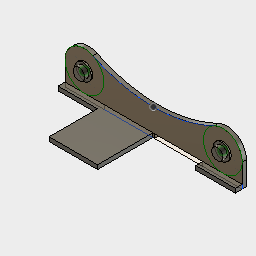
spoolholder (Autodesk Fusion 360 design; units mm, degrees)
Autodesk Fusion 360 part; units mm, degrees
sketch "Sketch1" plane through (0, 0, 0) normal (0, 0, 1) x (1, 0, 0)
  circle A0 centre (-50, 0) radius 4.1
  circle A1 centre (50, 0) radius 4.1
  circle A2 centre (50, 0) radius 14
  circle A3 centre (50, 0) radius 6
  circle A4 centre (-50, 0) radius 14
  circle A5 centre (-50, 0) radius 6
  line L0 (-64, -14) -> (64, -14)
  line L1 (-64, 0) -> (-64, -14)
  line L2 (64, 0) -> (64, -14)
  arc A6 (-43.8635, 12.5835) -> (43.8635, 12.5835) centre (0, 102.5297) ccw
  line L3 (-64, -14) -> (64, -14)
  line L4 (64, -14) -> (64, -17)
  line L5 (64, -17) -> (-64, -17)
  line L6 (-64, -17) -> (-64, -14)
  line L7 (0.5, -14) -> (35.5, -14)
  line L8 (35.5, -14) -> (35.5, -17)
  line L9 (35.5, -17) -> (0.5, -17)
  line L10 (0.5, -17) -> (0.5, -14)
  line L11 (-0.5, -14) -> (-35.5, -14)
  line L12 (-35.5, -14) -> (-35.5, -17)
  line L13 (-35.5, -17) -> (-0.5, -17)
  line L14 (-0.5, -17) -> (-0.5, -14)
  point P0 (-0.113, 2.4581)
  dimension "d1" = 8.2
  dimension "d2" = 8.2
  dimension "d3" = 50
  dimension "d4" = 50
  dimension "d5" = 28
  dimension "d6" = 12
  dimension "d7" = 28
  dimension "d8" = 12
  dimension "d9" = 14
  dimension "d10" = 3
  dimension "d11" = 3
  dimension "d12" = 35
  dimension "d13" = 35.5
  dimension "d20" = 35
  dimension "d21" = 35.5
  measures "d1" diameter of A0
  measures "d2" diameter of A1
  measures "d3" distance of origin A1.centre
  measures "d4" distance of origin A0.centre
  measures "d5" diameter of A2
  measures "d6" diameter of A3
  measures "d7" diameter of A4
  measures "d8" diameter of A5
  measures "d9" distance of A1.centre L0
  measures "d10" distance of L0.end L4.end
  measures "d11" distance of L7.start L9.end
  measures "d12" distance of L8.end L9.end
  measures "d13" distance of origin L8
  measures "d20" distance of L11.start L11.end
  measures "d21" distance of origin L12
extrude "Extrude1" add sketch "Sketch1" against normal blind 3 contours A0 | A1 | A2 | A2 L0 L2 L3 | A2 A4 L0 A6 L3 L7 L11 | L0 L3 L4 L5 L8 | A4 | A4 L0 L1 L3 | L0 L3 L5 L10 L14 | L0 L3 L5 L6 L12 | L0 L3 L5 L11 L12 L13 L14 | A3 | A5
extrude "Extrude2" add sketch "Sketch1" along normal blind 1 contours A3 | A5
extrude "Extrude3" add sketch "Sketch1" along normal blind 4 contours A0 | A1
extrude "Extrude4" add sketch "Sketch1" along normal blind 40 contours L0 L3 L5 L11 L12 L13 L14
extrude "Extrude5" add sketch "Sketch1" along normal blind 5 contours L0 L3 L4 L5 L8 | L0 L3 L5 L6 L12
